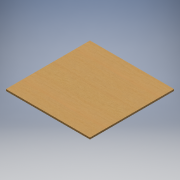
# Autodesk Inventor part: Floor
Saved by Autodesk Inventor 2019 (Build 230136000, 136)
## iProperties
Created: 2019-08-18
Part Number: Floor
Material: Generic
Document SubType Name: Modeling
Designer: Bruno
Density: 1 g/cm^3
Appearance: Default
Author: Bruno
Autodesk Inventor part; units mm, degrees
ref_plane "YZ Plane" through (0, 0, 0) normal (1, 0, 0) x (0, 1, 0)
ref_plane "XZ Plane" through (0, 0, 0) normal (0, 1, 0) x (-1, 0, 0)
ref_plane "XY Plane" through (0, 0, 0) normal (0, 0, 1) x (1, 0, 0)
sketch "Sketch1" plane through (0, 0, 0) normal (0, 1, 0) x (-1, 0, 0)
  line L0 (200, -200) -> (-200, -200)
  line L1 (-200, -200) -> (-200, 200)
  line L2 (-200, 200) -> (200, 200)
  line L3 (200, 200) -> (200, -200)
  line L4 (160, -160) -> (-160, -160) construction
  line L5 (-160, -160) -> (-160, 160) construction
  line L6 (-160, 160) -> (160, 160) construction
  line L7 (160, 160) -> (160, -160) construction
  line L8 (0, 42.2223) -> (0, -35.1237) construction
  line L9 (40.4991, 0) -> (-29.63, 0) construction
  point P0 (0, 0)
  dimension "d0" = 400
  dimension "d1" = 320
  dimension "d2" = 320
  dimension "d3" = 400
  constraints: 20 end point, 4 parallel, 3 horizontal, 2 perpendicular, 2 point on line, 1 vertical, 4 other
  measures "d0" distance of L0.start L0.end
  measures "d1" distance of L4.start L4.end
  measures "d2" distance of L6.end L4.start
  measures "d3" distance of L0.end L1.end
extrude "Extrusion1" add sketch "Sketch1" along normal blind 8
sketch "Sketch3" plane through (0, 8, 0) normal (0, 1, 0) x (1, 0, 0)
  circle A0 centre (-190, 190) radius 2.5
  circle A1 centre (-190, 160) radius 2.5
  line L0 (-190, 160) -> (-190, 190) construction
  line L1 (-200, 200) -> (-200, -200) projected
  line L2 (-200, 190) -> (-190, 190) construction
  line L3 (-190, 190) -> (-190, 200) construction
  line L4 (200, 200) -> (-200, 200) projected
  circle A2 centre (-190, -160) radius 2.5
  circle A3 centre (-190, -190) radius 2.5
  circle A4 centre (190, -160) radius 2.5
  circle A5 centre (190, -190) radius 2.5
  circle A6 centre (190, 190) radius 2.5
  circle A7 centre (190, 160) radius 2.5
  line L5 (-190, -160) -> (-190, -190) construction
  line L6 (190, -190) -> (190, -160) construction
  line L7 (190, 160) -> (190, 190) construction
  line L8 (-190, -190) -> (-190, -200) construction
  line L9 (-200, -200) -> (200, -200) projected
  line L10 (-190, -190) -> (-200, -190) construction
  line L11 (190, -190) -> (190, -200) construction
  line L12 (200, -200) -> (200, 200) projected
  line L13 (190, -190) -> (200, -190) construction
  line L14 (190, 190) -> (200, 190) construction
  line L15 (190, 190) -> (190, 200) construction
  point P0 (0, 0)
  dimension "d6" = 5
  dimension "d7" = 30
  dimension "d8" = 10
  dimension "d9" = 10
  constraints: 24 end point, 9 equal length, 8 centre point, 8 point on line, 7 equal radius, 6 vertical, 5 perpendicular, 1 horizontal
  measures "d6" diameter of A0
  measures "d7" distance of L0.start L0.end
  measures "d8" distance of L0.end L3.end
  measures "d9" distance of L2.start L0.end
extrude "Extrusion2" cut sketch "Sketch3" against normal through all contours A0 | A1 | A2 | A3 | A4 | A5 | A6 | A7
body "Solid1"
